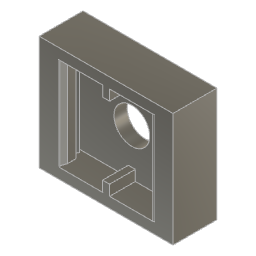
ECM Button Angle Supports v4 (Autodesk Fusion 360 archive; units mm, degrees)
design "PUSH BUTTON SUPPORT"
Autodesk Fusion 360 part; units mm, degrees
sketch "Sketch1" plane through (0, 0, 0) normal (0, 1, 0) x (1, 0, 0)
  line L0 (2.815, 2.25) -> (-2.815, 2.25)
  line L1 (-2.815, 2.25) -> (-2.815, -2.25)
  line L2 (-2.815, -2.25) -> (2.815, -2.25)
  line L3 (2.815, -2.25) -> (2.815, 2.25)
  line L4 (2.815, 2.25) -> (-2.815, -2.25) construction
  line L5 (-2.815, 2.25) -> (2.815, -2.25) construction
  line L6 (3.815, 3.25) -> (-3.815, 3.25)
  line L7 (-3.815, 3.25) -> (-3.815, -3.25)
  line L8 (-3.815, -3.25) -> (3.815, -3.25)
  line L9 (3.815, -3.25) -> (3.815, 3.25)
  line L10 (3.815, 3.25) -> (-3.815, -3.25) construction
  line L11 (-3.815, 3.25) -> (3.815, -3.25) construction
  line L12 (1, 1.85) -> (-1, 1.85)
  line L13 (1, 1.85) -> (-1, -1.85) construction
  line L14 (-1, 1.85) -> (1, -1.85) construction
  line L15 (-0.994265, -2.25) -> (1, -2.25)
  line L16 (1, -2.25) -> (1, -1.85)
  line L17 (1, -1.85) -> (-0.994265, -1.85)
  line L18 (-0.994265, -1.85) -> (-0.994265, -2.25)
  line L19 (1, 1.85) -> (1, 2.25)
  line L20 (1, 2.25) -> (-1, 2.25)
  line L21 (-1, 2.25) -> (-1, 1.85)
  line L22 (-2.815, -2.25) -> (-2.515, -2.25)
  line L23 (-2.515, -2.25) -> (-2.515, 2.25)
  line L24 (-2.515, 2.25) -> (-2.815, 2.25)
  line L25 (-2.815, 2.25) -> (-2.815, -2.25)
  line L26 (2.815, -2.25) -> (2.515, -2.25)
  line L27 (2.515, -2.25) -> (2.515, 2.25)
  line L28 (2.515, 2.25) -> (2.815, 2.25)
  line L29 (2.815, 2.25) -> (2.815, -2.25)
  dimension "d1" = 5.63
  dimension "d2" = 4.5
  dimension "d3" = 7.63
  dimension "d4" = 6.5
  dimension "d7" = 2
  dimension "d8" = 3.7
  dimension "d11" = 0.3
  dimension "d12" = 0.3
  constraint horizontal L0
  constraint perpendicular L0 L1
  constraint parallel L0 L2
  constraint parallel L1 L3
  constraint coincident L4 origin
  constraint coincident L5 origin
  constraint horizontal L6
  constraint perpendicular L6 L7
  constraint parallel L6 L8
  constraint parallel L7 L9
  constraint coincident L10 origin
  constraint coincident L11 origin
  constraint horizontal L12
  constraint coincident L13 origin
  constraint coincident L14 origin
  constraint horizontal L15
  constraint vertical L16
  constraint horizontal L17
  constraint vertical L18
  constraint vertical L19
  constraint horizontal L20
  constraint vertical L21
  constraint coincident L0 L19.end
  constraint horizontal L22
  constraint vertical L23
  constraint horizontal L24
  constraint vertical L25
  constraint horizontal L26
  constraint vertical L27
  constraint horizontal L28
  constraint vertical L29
  measures "d1" distance of L1.end L2.end
  measures "d2" distance of L0.end L1.end
  measures "d3" distance of L7.end L8.end
  measures "d4" distance of L6.end L7.end
  measures "d7" distance of L13.end L14.end
  measures "d8" distance of L12.end L13.end
  measures "d11" distance of L1.end L22.end
  measures "d12" distance of L2.end L26.end
extrude "Extrude1" add sketch "Sketch1" along normal blind 5 contours L6 L7 L8 L9 picked at (-0.331422, -2.916667)
extrude "Extrude2" add sketch "Sketch1" along normal blind 5 contours L0 L12 L19 L20 L21 | L2 L15 L16 L17 L18 picked at (-0.333333, 2.116667) picked at (0.335245, -2.116667)
extrude "Extrude3" add sketch "Sketch1" along normal blind 1.8 contours L0 L2 L3 L26 L27 L28 L29 | L0 L1 L2 L22 L23 L24 L25 picked at (2.615, 0.75) picked at (-2.715, 0.75)
chamfer "Chamfer1" distance 0.3 angle 45 2 edges at (-2.515, 1.8, 0) (2.515, 1.8, 0)
chamfer "Chamfer3" distance 0.9 distance2 0.3 1 edges at (-2.515, 0, 0) measured on face at (-2.515, 0.50002, 0.75)
chamfer "Chamfer4" distance 0.3 distance2 1 1 edges at (2.515, 0, 0) measured on face at (3.381667, 0, 0.75)
sketch "Sketch2" plane through (0, 0, 3.25) normal (0, 0, 1) x (-1, 0, 0)
  line L0 (3.815, 0) -> (-3.815, 0)
  line L1 (-3.815, 0) -> (-3.815, -5)
  line L2 (-3.815, -5) -> (3.815, -5)
  line L3 (3.815, -5) -> (3.815, 0)
  line L4 (-2.81825, -1.967525) -> (2.836671, -1.967525)
  line L5 (2.836671, -1.967525) -> (2.836671, -2.718821)
  line L6 (2.836671, -2.718821) -> (-2.81825, -2.718821)
  line L7 (-2.81825, -2.718821) -> (-2.81825, -1.967525)
  constraint horizontal L4
  constraint vertical L5
  constraint horizontal L6
  constraint vertical L7
extrude "Extrude4" add sketch "Sketch2" against normal blind 6.5 contours L4 L5 L6 L7 picked at (-0.933276, -2.217957)
sketch "Sketch3" plane through (0, 1.967525, 0) normal (0, -1, 0) x (1, 0, 0)
  line L0 (-1, -1.85) -> (1, -1.85)
  line L1 (1, -1.85) -> (1, -2.25)
  line L2 (1, -2.25) -> (2.815, -2.25)
  line L3 (2.815, -2.25) -> (2.815, 2.25)
  line L4 (2.815, 2.25) -> (1, 2.25)
  line L5 (1, 2.25) -> (1, 1.85)
  line L6 (1, 1.85) -> (-0.994265, 1.85)
  line L7 (-0.994265, 1.85) -> (-0.994265, 2.25)
  line L8 (-0.994265, 2.25) -> (-2.815, 2.25)
  line L9 (-2.815, 2.25) -> (-2.815, -2.25)
  line L10 (-2.815, -2.25) -> (-1, -2.25)
  line L11 (-1, -2.25) -> (-1, -1.85)
  circle A0 centre (0, 0) radius 1.019835
  constraint coincident A0.centre origin
extrude "Extrude5" cut sketch "Sketch3" against normal blind 6.5 contours A0 picked at (-0.371624, 0.422719)
extrude "Extrude6" cut 1 faces at (-0.331422, 5, 2.916667) along direction (0, -1, 0) blind 2
extrude "Extrude7" cut 1 faces at (1, 0.655842, -1.983333) along direction (-1, 0, 0) blind 0.3
extrude "Extrude8" cut 1 faces at (1, 0.655842, 2.116667) along direction (-1, 0, 0) blind 0.3
extrude "Extrude9" cut 1 faces at (-1, 0.655842, -2.116667) along direction (1, 0, 0) blind 0.3
extrude "Extrude10" cut 1 faces at (-0.994265, 0.655842, 1.983333) along direction (1, 0, 0) blind 0.3
extrude "Extrude11" cut 2 faces at (-1.305, 0.955842, -2.25) (1.305, 0.989175, -2.25) along direction (0, 0, -1) blind 0.3
extrude "Extrude12" cut 2 faces at (-1.301176, 0.955842, 2.25) (1.305, 0.989175, 2.25) along direction (0, 0, 1) blind 0.3
extrude "Extrude13" cut 1 faces at (-3.481667, 0, -0.85) along direction (0, 1, 0) blind 0.5
extrude "Extrude14" cut 1 faces at (-2.815, 0.166667, -0.85) along direction (1, 0, 0) blind 8
extrude "Extrude15" cut 2 faces at (2.81498, 1.8, 0.85) (2.71496, 1.70002, -0.85) along direction (0.70710678, -0.70710678, 0) blind 0.3
extrude "Extrude16" cut 2 faces at (-2.81498, 1.8, -0.85) (-2.71496, 1.70002, -0.85) along direction (-0.70710678, -0.70710678, 0) blind 0.3
extrude "Extrude17" cut 1 faces at (2.565, 0.833333, 0.85) along direction (0.95782629, 0.28734789, 0) blind 0.1
extrude "Extrude18" cut 1 faces at (-2.559444, 0.766667, 0.85) along direction (-0.9486833, 0.31622777, 0) blind 0.1
extrude "Extrude19" cut 1 faces at (2.515, 1.166687, 0.85) along direction (1, 0, 0) blind 0.1
extrude "Extrude20" cut 1 faces at (-2.515, 1.10002, 0.85) along direction (-1, 0, 0) blind 0.1
extrude "Extrude21" cut 1 faces at (-2.815, 1.911683, -0.85) along direction (-1, 0, 0) blind 0.2
extrude "Extrude22" cut 1 faces at (2.815, 1.911683, -0.85) along direction (1, 0, 0) blind 0.2
extrude "Extrude23" cut 1 faces at (-0.7, 0.989175, -2.316667) along direction (1, 0, 0) blind 0.5
extrude "Extrude24" cut 1 faces at (-0.694265, 1.47835, 2.316667) along direction (1, 0, 0) blind 0.5
extrude "Extrude25" cut 1 faces at (0.7, 0.989175, 2.316667) along direction (-1, 0, 0) blind 0.5
extrude "Extrude26" cut 1 faces at (0.7, 1.47835, -2.316667) along direction (-1, 0, 0) blind 0.5
extrude "Extrude27" cut 1 faces at (0.068578, 0.989175, 1.85) along direction (0, 0, 1) blind 0.2
extrude "Extrude28" cut 1 faces at (0.066667, 0.989175, -1.85) along direction (0, 0, -1) blind 0.2
extrude "Extrude29" cut 2 faces at (1.005, 1.289195, -2.55) (-1.005, 1.289195, -2.55) along direction (0, 0, -1) blind 0.1
extrude "Extrude30" cut 2 faces at (-1.001176, 1.289195, 2.55) (1.005, 1.289195, 2.55) along direction (0, 0, 1) blind 0.1
chamfer "Chamfer2" [suppressed]
